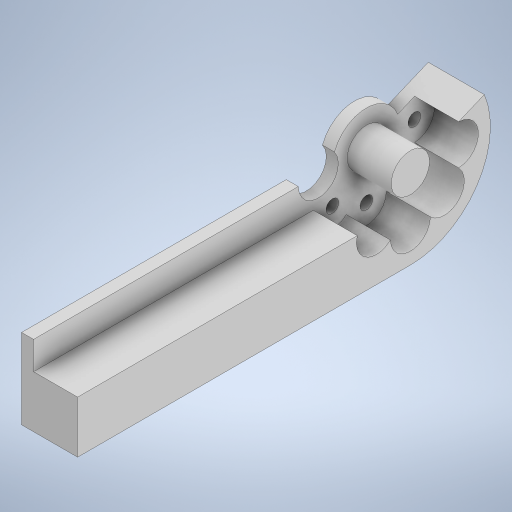
# Autodesk Inventor part: toe_springjoinbace_under_left
Saved by Autodesk Inventor 2024.1 (Build 281209000, 209)
## iProperties
Created: 2024-02-25
Part Number: toe_springjoinbace_under_left
Material: 一般
Document SubType Name: Modeling
Designer: hibik
Density: 1 g/cm^3
Appearance: 既定
Author: hibik
Autodesk Inventor part; units mm, degrees
ref_plane "YZ Plane" through (0, 0, 0) normal (1, 0, 0) x (0, 1, 0)
ref_plane "XZ Plane" through (0, 0, 0) normal (0, 1, 0) x (-1, 0, 0)
ref_plane "XY Plane" through (0, 0, 0) normal (0, 0, 1) x (1, 0, 0)
sketch "スケッチ1" plane through (0, 0, 0) normal (1, 0, 0) x (0, 1, 0)
  circle A0 centre (0, 0) radius 4.25
  circle A1 centre (0, 0) radius 6 construction
  circle A2 centre (6, 0) radius 0.8
  line L0 (-14, 0) -> (14, 0) projected
  circle A3 centre (4.2426, 4.2426) radius 0.8
  circle A4 centre (0, 6) radius 0.8
  circle A5 centre (-4.2426, 4.2426) radius 0.8
  circle A6 centre (-6, 0) radius 0.8
  circle A7 centre (-4.2426, -4.2426) radius 0.8
  circle A8 centre (0, -6) radius 0.8
  circle A9 centre (4.2426, -4.2426) radius 0.8
  circle A10 centre (0, 0) radius 2.4
  line L1 (0, 0) -> (0, 6)
  line L2 (0, 0) -> (2.2961, -5.5433)
  circle A11 centre (0, 0) radius 10
  line L3 (2.2961, -5.5433) -> (3.8268, -9.2388)
  line L4 (0, -9.2388) -> (-10, -9.2388)
  line L5 (-10, -9.2388) -> (-10, 41.5747)
  line L6 (-10, 41.5747) -> (0, 41.5747)
  line L7 (0, 41.5747) -> (0, -9.2388)
  line L8 (0, -6) -> (4.2426, -4.2426) construction
  line L9 (0, -9.2388) -> (3.8268, -9.2388)
  circle A12 centre (0, 6) radius 2.5
  point P0 (0, 5.2)
  point P1 (0, 6.8)
  point P2 (-10, 0)
  point P3 (2.1213, -5.1213)
  point P4 (0, 2.4)
  point P5 (0.9184, -2.2173)
  point P6 (1.4789, 3.9844)
  point P7 (0, 8.5)
  point P8 (1.6264, -3.9265)
  dimension "d0" = 8.5
  dimension "d1" = 12
  dimension "d2" = 1.6
  dimension "d5" = 360
  dimension "d7" = 4.8
  dimension "d8" = 4
  dimension "d21" = 5
  constraints: 18 end point, 12 centre point, 6 coincident, 6 point on line, 3 point on circle, 2 horizontal, 2 parallel, 1 midpoint, 1 perpendicular, 1 vertical, 20 other
  measures "d0" diameter of A0
  measures "d1" diameter of A1
  measures "d2" diameter of A2
  measures "d7" diameter of A10
  measures "d21" diameter of A12
extrude "押し出し1" add sketch "スケッチ1" along normal blind 1.5 contours L0 A10 L1 A12 A0 | A0 L2 A10 L0 | L2 L3 L9 L7 A8 A0 | A0 L7 A10 L2 | A10 L2 L0 | L0 L1 A10 | L1 A10 L0 A0 A12 | L7 A8 L4 A11 L0 A6 A0 | A0 L0 A10 L7 | A10 L7 L2 | L7 A10 L0 | L0 A10 L1 | A0 L0 A6 A11 L7 A12 | A11 L4 L9 | A11 L5 L6 L7
sketch "スケッチ3" plane through (1.5, 0, 0) normal (1, 0, 0) x (0, 0, -1)
  circle A0 centre (0, 0) radius 2.5 construction
  line L0 (0, -2.5) -> (-41.5747, -2.5) construction
  line L1 (-41.5747, -2.5) -> (0, -2.5)
  line L2 (0, -2.5) -> (0, -3.5)
  line L3 (0, -3.5) -> (-41.5747, -3.5)
  line L4 (-41.5747, -3.5) -> (-41.5747, -2.5)
  circle A1 centre (0, 0) radius 3.5
  line L5 (-41.5747, 0) -> (-41.5747, -10) projected
  line L6 (-8.5, 0) -> (-41.5747, 0) projected
  line L7 (-41.5747, 0) -> (-41.5747, -10) projected
  line L8 (-41.5747, -10) -> (0, -10) projected
  arc A2 (0, -10) -> (9.2388, 3.8268) centre (0, 0) ccw projected
  line L9 (9.2388, 3.8268) -> (3.9265, 1.6264) projected
  circle A3 centre (4.2426, -4.2426) radius 0.8 projected
  circle A4 centre (-4.2426, -4.2426) radius 0.8 projected
  circle A5 centre (0, -6) radius 0.8 projected
  circle A6 centre (-4.2426, -4.2426) radius 2.5
  circle A7 centre (0, -6) radius 2.5
  circle A8 centre (4.2426, -4.2426) radius 2.5
  circle A9 centre (6, 0) radius 0.8 projected
  circle A10 centre (6, 0) radius 2.5
  arc A11 (-8.5, 0) -> (-3.9844, 1.4789) centre (-6, 0) ccw projected
  arc A12 (3.9265, 1.6264) -> (-3.9844, 1.4789) centre (0, 0) ccw projected
  circle A13 centre (0, 0) radius 2.4
  point P0 (6.0349, 2.4998)
  point P1 (6.0349, -2.4998)
  point P2 (2.4998, -6.0349)
  point P3 (-2.4998, -6.0349)
  point P4 (-6.6298, -3.5)
  dimension "d13" = 5
  dimension "d14" = 1
  dimension "d15" = 5
  dimension "d16" = 5
  dimension "d17" = 5
  dimension "d18" = 5
  dimension "d22" = 4.8
  constraints: 10 end point, 8 coincident, 6 centre point, 3 horizontal, 2 parallel, 1 collinear, 1 perpendicular, 1 point on line, 1 tangent, 1 vertical alignment, 2 other
  measures "d14" distance between parallel lines of L0 L3
  measures "d15" diameter of A6
  measures "d16" diameter of A7
  measures "d17" diameter of A8
  measures "d18" diameter of A10
  measures "d22" diameter of A13
extrude "押し出し2" add sketch "スケッチ3" along normal blind 5.5 contours L3 A6 A7 A8 A10 L9 A2 L8 L5 | A13
